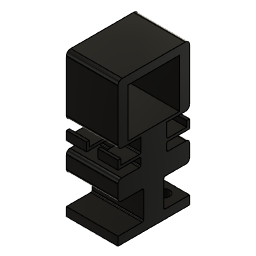
Управляющая голова конвейер v7 (Autodesk Fusion 360 design; units mm, degrees)
Autodesk Fusion 360 part; units mm, degrees
sketch "Sketch1" plane through (0, 0, 0) normal (1, 0, 0) x (0, 0, -1)
  line L0 (0, 0) -> (-18, 0)
  line L1 (-18, 0) -> (-18, 17)
  line L2 (-18, 17) -> (0, 17)
  line L3 (0, 17) -> (0, 0)
  line L4 (-21.5, 20) -> (3.5, 20)
  line L5 (3.5, 20) -> (3.5, -30)
  line L6 (3.5, -30) -> (-21.5, -30)
  line L7 (-21.5, -30) -> (-21.5, 20)
  dimension "d1" = 18
  dimension "d2" = 17
  dimension "d3" = 25
  dimension "d4" = 50
  dimension "d66" = 3.5
  constraint horizontal L0
  constraint vertical L1
  constraint horizontal L2
  constraint vertical L3
  constraint coincident L0.start L3.end
  constraint horizontal L4
  constraint vertical L5
  constraint horizontal L6
  constraint vertical L7
  measures "d1" distance of L0.start L0.end
  measures "d2" distance of L0.start L2.end
  measures "d3" distance of L4.start L4.end
  measures "d4" distance of L4.start L6.end
  measures "d66" distance of L3 L5
extrude "Extrude1" add sketch "Sketch1" against normal blind 18
fillet "Fillet1" radius 1.5 2 edges at (-9, 20, -3.5) (-9, 20, 21.5)
sketch "Sketch2" plane through (0, 0, 0) normal (1, 0, 0) x (0, 0, -1)
  line L0 (-18, 17) -> (0, 17)
  line L1 (0, 17) -> (0, 0)
  line L2 (0, 0) -> (-18, 0)
  line L3 (-18, 0) -> (-18, 17)
  arc A0 (-20, 20) -> (-21.5, 18.5) centre (-20, 18.5) ccw
  line L4 (-21.5, 18.5) -> (-21.5, -30)
  line L5 (-21.5, -30) -> (3.5, -30)
  line L6 (3.5, -30) -> (3.5, 18.5)
  arc A1 (3.5, 18.5) -> (2, 20) centre (2, 18.5) ccw
  line L7 (2, 20) -> (-20, 20)
  line L8 (-21.5, -3.9907) -> (-20.5, -3.9907)
  line L9 (-20.5, -3.9907) -> (-20.5, -6)
  line L10 (-20.5, -6) -> (-13.5, -6)
  line L11 (-13.5, -6) -> (-13.5, -0.9907)
  line L12 (-13.5, -0.9907) -> (-21.5, -0.9907)
  line L13 (3.5, -1) -> (-4.5, -1)
  line L14 (-4.5, -1) -> (-4.5, -6)
  line L15 (-4.5, -6) -> (2.5, -6)
  line L16 (2.5, -6) -> (2.5, -4)
  line L17 (2.5, -4) -> (3.5, -4)
  dimension "d9" = 7
  dimension "d10" = 8
  dimension "d12" = 5.0093
  dimension "d13" = 1
  dimension "d14" = 3
  dimension "d15" = 3
  dimension "d16" = 5
  dimension "d17" = 1
  constraint coincident L4 L8.start
  constraint perpendicular L4 L8
  constraint perpendicular L8 L9
  constraint perpendicular L9 L10
  constraint perpendicular L2 L11
  constraint coincident L4 L12.end
  constraint perpendicular L4 L12
  constraint coincident L6 L13.start
  constraint perpendicular L6 L13
  constraint perpendicular L12 L14
  constraint perpendicular L6 L15
  constraint perpendicular L15 L16
  constraint coincident L6 L17.end
  constraint perpendicular L6 L17
  measures "d9" distance of L9.end L10.end
  measures "d10" distance of L13.start L13.end
  measures "d12" distance of L10 L12
  measures "d13" distance of L8.start L8.end
  measures "d14" distance of L8 L12
  measures "d15" distance of L13 L17
  measures "d16" distance of L13 L15
  measures "d17" distance of L16.end L17.end
extrude "Extrude2" cut sketch "Sketch2" against normal blind 43 contours L4 L8 L9 L10 L11 L12 | L6 L13 L14 L15 L16 L17
sketch "Sketch3" plane through (0, 0, 21.5) normal (0, 0, 1) x (1, 0, 0)
  line L0 (0, -3.9907) -> (-18, -3.9907)
  line L1 (-18, -3.9907) -> (-18, -30)
  line L2 (-18, -30) -> (0, -30)
  line L3 (0, -30) -> (0, -3.9907)
  line L4 (0, -3.9907) -> (-7, -3.9907)
  line L5 (-7, -3.9907) -> (-7, -5.9907)
  line L6 (-7, -5.9907) -> (0, -5.9907)
  line L7 (0, -5.9907) -> (0, -3.9907)
  line L8 (-18, -3.9907) -> (-11, -3.9907)
  line L9 (-11, -3.9907) -> (-11, -5.9907)
  line L10 (-11, -5.9907) -> (-18, -5.9907)
  line L11 (-18, -5.9907) -> (-18, -3.9907)
  line L12 (-11, -3.9907) -> (-7, -3.9907)
  line L13 (-7, -3.9907) -> (-7, -5.9907)
  line L14 (-7, -5.9907) -> (-11, -5.9907)
  line L15 (-11, -5.9907) -> (-11, -3.9907)
  dimension "d21" = 7
  dimension "d22" = 2
  dimension "d23" = 7
  dimension "d24" = 2
  constraint horizontal L4
  constraint vertical L5
  constraint horizontal L6
  constraint vertical L7
  constraint coincident L0.start L3.end
  constraint horizontal L8
  constraint vertical L9
  constraint horizontal L10
  constraint vertical L11
  constraint coincident L0.end L1.start
  constraint horizontal L12
  constraint vertical L13
  constraint horizontal L14
  constraint vertical L15
  measures "d21" distance of L0.start L4.end
  measures "d22" distance of L0.start L6.end
  measures "d23" distance of L0.end L8.end
  measures "d24" distance of L8 L10
extrude "Extrude3" cut sketch "Sketch3" against normal blind 8 contours L0 L5 L9 L12 L13 L14 L15
sketch "Sketch4" plane through (0, 0, -3.5) normal (0, 0, -1) x (-1, 0, 0)
  line L0 (18, -4) -> (0, -4)
  line L1 (0, -4) -> (0, -30)
  line L2 (0, -30) -> (18, -30)
  line L3 (18, -30) -> (18, -4)
  line L4 (0, -4) -> (7, -4)
  line L5 (7, -4) -> (7, -6)
  line L6 (7, -6) -> (0, -6)
  line L7 (0, -6) -> (0, -4)
  line L8 (18, -4) -> (11, -4)
  line L9 (11, -4) -> (11, -6)
  line L10 (11, -6) -> (18, -6)
  line L11 (18, -6) -> (18, -4)
  line L12 (7, -4) -> (11, -4)
  line L13 (11, -4) -> (11, -6)
  line L14 (11, -6) -> (7, -6)
  line L15 (7, -6) -> (7, -4)
  dimension "d27" = 7
  dimension "d28" = 2
  dimension "d29" = 7
  dimension "d30" = 2
  constraint horizontal L4
  constraint vertical L5
  constraint horizontal L6
  constraint vertical L7
  constraint coincident L0.end L1.start
  constraint horizontal L8
  constraint vertical L9
  constraint horizontal L10
  constraint vertical L11
  constraint coincident L0.start L3.end
  constraint horizontal L12
  constraint vertical L13
  constraint horizontal L14
  constraint vertical L15
  measures "d27" distance of L0.end L4.end
  measures "d28" distance of L0.end L6.end
  measures "d29" distance of L0.start L8.end
  measures "d30" distance of L0.start L10.end
extrude "Extrude4" cut sketch "Sketch4" against normal blind 8 contours L0 L5 L9 L12 L13 L14 L15
sketch "Sketch5" plane through (0, 0, -3.5) normal (0, 0, -1) x (-1, 0, 0)
  line L0 (7, -6) -> (7, -4)
  line L1 (7, -4) -> (0, -4)
  line L2 (0, -4) -> (0, -30)
  line L3 (0, -30) -> (18, -30)
  line L4 (18, -30) -> (18, -4)
  line L5 (18, -4) -> (11, -4)
  line L6 (11, -4) -> (11, -6)
  line L7 (11, -6) -> (7, -6)
  line L8 (7, -4) -> (11, -4)
  line L9 (11, -4) -> (11, -10)
  line L10 (11, -10) -> (7, -10)
  line L11 (7, -10) -> (7, -4)
  line L12 (11, -10) -> (18, -10)
  line L13 (18, -10) -> (18, -7)
  line L14 (18, -7) -> (11, -7)
  line L15 (11, -7) -> (11, -10)
  line L16 (7, -10) -> (0, -10)
  line L17 (0, -10) -> (0, -7)
  line L18 (0, -7) -> (7, -7)
  line L19 (7, -7) -> (7, -10)
  dimension "d33" = 3
  constraint horizontal L8
  constraint vertical L9
  constraint horizontal L10
  constraint vertical L11
  constraint coincident L0.end L1.start
  constraint horizontal L12
  constraint vertical L13
  constraint horizontal L14
  constraint vertical L15
  constraint horizontal L16
  constraint vertical L17
  constraint horizontal L18
  constraint vertical L19
  constraint coincident L2 L17.end
  measures "d33" distance of L9.end L14.end
extrude "Extrude5" cut sketch "Sketch5" against normal blind 8 contours L0 L6 L7 L8 L9 L11 | L7 L9 L10 L11 L15 L19 | L2 L11 L16 L17 L18 L19 | L4 L9 L12 L13 L14 L15
sketch "Sketch6" plane through (0, 0, 21.5) normal (0, 0, 1) x (1, 0, 0)
  line L0 (-11, -5.9907) -> (-11, -3.9907)
  line L1 (-11, -3.9907) -> (-18, -3.9907)
  line L2 (-18, -3.9907) -> (-18, -30)
  line L3 (-18, -30) -> (0, -30)
  line L4 (0, -30) -> (0, -3.9907)
  line L5 (0, -3.9907) -> (-7, -3.9907)
  line L6 (-7, -3.9907) -> (-7, -5.9907)
  line L7 (-7, -5.9907) -> (-11, -5.9907)
  line L8 (-11, -5.9907) -> (-7, -5.9907)
  line L9 (-7, -5.9907) -> (-7, -9.9907)
  line L10 (-7, -9.9907) -> (-11, -9.9907)
  line L11 (-11, -9.9907) -> (-11, -5.9907)
  line L12 (-7, -9.9907) -> (0, -9.9907)
  line L13 (0, -9.9907) -> (0, -6.9907)
  line L14 (0, -6.9907) -> (-7, -6.9907)
  line L15 (-7, -6.9907) -> (-7, -9.9907)
  line L16 (-11, -9.9907) -> (-18, -9.9907)
  line L17 (-18, -9.9907) -> (-18, -6.9907)
  line L18 (-18, -6.9907) -> (-11, -6.9907)
  line L19 (-11, -6.9907) -> (-11, -9.9907)
  dimension "d36" = 4
  dimension "d37" = 3
  dimension "d38" = 3
  dimension "d39" = 7
  constraint horizontal L8
  constraint vertical L9
  constraint horizontal L10
  constraint vertical L11
  constraint coincident L0.start L7.end
  constraint horizontal L12
  constraint vertical L13
  constraint horizontal L14
  constraint vertical L15
  constraint horizontal L16
  constraint vertical L17
  constraint horizontal L18
  constraint vertical L19
  measures "d36" distance of L0.start L10.end
  measures "d37" distance of L9.end L14.end
  measures "d38" distance of L10.end L18.end
  measures "d39" distance of L13 L15
extrude "Extrude6" cut sketch "Sketch6" against normal blind 8 contours L7 L8 L9 L10 L11 L15 L19 | L2 L11 L16 L17 L18 L19 | L4 L9 L12 L13 L14 L15
sketch "Sketch7" plane through (0, -30, 0) normal (0, -1, 0) x (1, 0, 0)
  line L0 (0, -3.5) -> (0, 21.5)
  line L1 (0, 21.5) -> (-18, 21.5)
  line L2 (-18, 21.5) -> (-18, -3.5)
  line L3 (-18, -3.5) -> (0, -3.5)
sketch "Sketch8" plane through (0, 0, 0) normal (1, 0, 0) x (0, 0, -1)
  line L0 (-13.5, -9.9907) -> (-21.5, -9.9907)
  line L1 (-21.5, -9.9907) -> (-21.5, -30)
  line L2 (-21.5, -30) -> (3.5, -30)
  line L3 (3.5, -30) -> (3.5, -10)
  line L4 (3.5, -10) -> (-4.5, -10)
  line L5 (-4.5, -10) -> (-4.5, -7)
  line L6 (-4.5, -7) -> (3.5, -7)
  line L7 (3.5, -7) -> (3.5, -4)
  line L8 (3.5, -4) -> (2.5, -4)
  line L9 (2.5, -4) -> (2.5, -6)
  line L10 (2.5, -6) -> (-4.5, -6)
  line L11 (-4.5, -6) -> (-4.5, -1)
  line L12 (-4.5, -1) -> (3.5, -1)
  line L13 (3.5, -1) -> (3.5, 18.5)
  arc A0 (3.5, 18.5) -> (2, 20) centre (2, 18.5) ccw
  line L14 (2, 20) -> (-20, 20)
  arc A1 (-20, 20) -> (-21.5, 18.5) centre (-20, 18.5) ccw
  line L15 (-21.5, 18.5) -> (-21.5, -0.9907)
  line L16 (-21.5, -0.9907) -> (-13.5, -0.9907)
  line L17 (-13.5, -0.9907) -> (-13.5, -6)
  line L18 (-13.5, -6) -> (-20.5, -6)
  line L19 (-20.5, -6) -> (-20.5, -3.9907)
  line L20 (-20.5, -3.9907) -> (-21.5, -3.9907)
  line L21 (-21.5, -3.9907) -> (-21.5, -6.9907)
  line L22 (-21.5, -6.9907) -> (-13.5, -6.9907)
  line L23 (-13.5, -6.9907) -> (-13.5, -9.9907)
  line L24 (-18, 17) -> (0, 17)
  line L25 (0, 17) -> (0, 0)
  line L26 (0, 0) -> (-18, 0)
  line L27 (-18, 0) -> (-18, 17)
  line L28 (-21.5, -30) -> (3.5, -30)
  line L29 (3.5, -30) -> (3.5, -27)
  line L30 (3.5, -27) -> (-21.5, -27)
  line L31 (-21.5, -27) -> (-21.5, -30)
  line L32 (-21.5, -27) -> (-12.5, -27)
  line L33 (-12.5, -27) -> (-12.5, -23)
  line L34 (-12.5, -23) -> (-21.5, -23)
  line L35 (-21.5, -23) -> (-21.5, -27)
  line L36 (3.5, -27) -> (-5.5, -27)
  line L37 (-5.5, -27) -> (-5.5, -23)
  line L38 (-5.5, -23) -> (3.5, -23)
  line L39 (3.5, -23) -> (3.5, -27)
  dimension "d42" = 3
  constraint horizontal L28
  constraint vertical L29
  constraint horizontal L30
  constraint vertical L31
  constraint coincident L1.end L2.start
  constraint horizontal L32
  constraint vertical L33
  constraint horizontal L34
  constraint vertical L35
  constraint horizontal L36
  constraint vertical L37
  constraint horizontal L38
  constraint vertical L39
  measures "d42" distance of L1.end L30.end
extrude "Extrude7" cut sketch "Sketch8" against normal blind 32 contours L1 L30 L32 L33 L34 L35 | L3 L30 L36 L37 L38 L39
fillet "Fillet2" radius 0.5 8 edges at (-14.5, -6, 13.5) (-3.5, -6, 13.5) (-3.5, -6.9907, 13.5) (-14.5, -6.9907, 13.5) (-3.5, -7, 4.5) (-3.5, -6, 4.5) (-14.5, -6, 4.5) (-14.5, -7, 4.5)
sketch "Sketch9" plane through (0, -30, 0) normal (0, -1, 0) x (1, 0, 0)
  line L0 (0, 20) -> (-18, 20)
  line L1 (-18, 20) -> (-18, -5)
  line L2 (-18, -5) -> (0, -5)
  line L3 (0, -5) -> (0, 20)
  line L4 (0, 20) -> (0, 7.5)
  line L5 (0, 7.5) -> (-18, 7.5)
  line L6 (-18, 7.5) -> (-13, 7.5)
  circle A0 centre (-13, 0.5) radius 2
  line L7 (-9, -5) -> (-9, 20)
  circle A1 centre (-5, 0.5) radius 2
  dimension "d50" = 4
  dimension "d63" = 4
  dimension "d64" = 4
  dimension "d65" = 4
  constraint horizontal L0
  constraint vertical L1
  constraint horizontal L2
  constraint vertical L3
  constraint midpoint L3 L4.end
  constraint midpoint L1 L5.end
  constraint coincident L5 L6.end
  constraint perpendicular L1 L6
  constraint midpoint L2 L7.start
  constraint midpoint L0 L7.end
  measures "d50" diameter of A0
  measures "d63" distance of A0.centre L7
  measures "d64" diameter of A1
  measures "d65" distance of L7 A1.centre
extrude "Extrude8" cut sketch "Sketch9" against normal blind 5 contours A0 | A1
extrude "Extrude9" cut 2 faces at (-12, -23, 15.5) (-12, -23, -0.5) along direction (0, 1, 0) blind 6
fillet "Fillet3" radius 1.25 4 edges at (-9, -9.9907, 21.5) (-9, -17, 21.5) (-9, -10, -3.5) (-9, -17, -3.5)
fillet "Fillet4" radius 0.5 4 edges at (-9, -10, 4.5) (-9, -17, 5.5) (-9, -17, 12.5) (-9, -9.9907, 13.5)
fillet "Fillet5" radius 0.5 2 edges at (-9, -27, 12.5) (-9, -27, 5.5)
fillet "Fillet6" radius 1.5 2 edges at (-9, -1, -3.5) (-9, -0.9907, 21.5)
